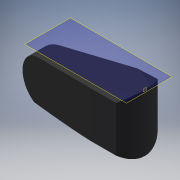
# Autodesk Inventor part: Sample Euph
Saved by Autodesk Inventor 2018 (Build 220112000, 112)
## iProperties
Created: 2018-02-07
Part Number: Sample Euph
Material: Generic
Document SubType Name: Modeling
Designer: owner
Density: 1 g/cm^3
Appearance: Default
Author: owner
Autodesk Inventor part; units mm, degrees
ref_plane "YZ Plane" through (0, 0, 0) normal (1, 0, 0) x (0, 1, 0)
ref_plane "XZ Plane" through (0, 0, 0) normal (0, 1, 0) x (-1, 0, 0)
ref_plane "XY Plane" through (0, 0, 0) normal (0, 0, 1) x (1, 0, 0)
sketch "Sketch1" plane through (0, 0, 0) normal (0, 0, 1) x (1, 0, 0)
  line L0 (171.45, 0) -> (908.05, 0)
  line L1 (0, 0) -> (908.05, 0) construction
  line L2 (908.05, 0) -> (908.05, 457.2)
  arc A0 (145.6057, 340.9409) -> (171.45, 0) centre (171.45, 171.45) ccw
  line L3 (908.05, 457.2) -> (145.6057, 340.9409)
  dimension "d0" = 908.05
  dimension "d2" = 457.2
  dimension "d6" = 342.9
  constraints: 8 end point, 2 horizontal, 2 point on circle, 1 centre point, 1 perpendicular, 1 point on line, 1 tangent
  measures "d0" distance of L1.start L0.end
  measures "d2" distance of L0.end L2.end
  measures "d6" diameter of A0
extrude "Extrusion1" add sketch "Sketch1" against normal blind 330.2
ref_plane "Work Plane1" through (171.45, 473.075, 0) normal (0, -1, 0) x (1, 0, 0)
sketch "Sketch2" plane through (171.45, 473.075, 0) normal (0, -1, 0) x (1, 0, 0)
  line L0 (-171.45, -101.6) -> (466.725, 0)
  line L1 (-171.45, 0) -> (0, 0) projected
  line L2 (-171.45, -101.6) -> (-222.6023, -185.7168)
  line L3 (-222.6023, -185.7168) -> (-171.45, -228.6)
  line L4 (-171.45, -330.2) -> (0, -330.2) projected
  line L5 (-171.45, -330.2) -> (-272.7707, -143.6584)
  line L6 (-272.7707, -143.6584) -> (-171.45, 0)
  line L7 (736.6, 0) -> (736.6, -330.2) projected
  arc A0 (673.1, -330.2) -> (673.1, 0) centre (490.22, -165.1) ccw
  line L8 (-171.45, -228.6) -> (673.1, -330.2)
  line L9 (0, -330.2) -> (732.1184, -387.4806)
  line L10 (732.1184, -387.4806) -> (736.6, -330.2)
  line L11 (0, 0) -> (704.85, 102.8193)
  line L12 (704.85, 102.8193) -> (736.6, 0)
  line L13 (466.725, 0) -> (673.1, 0)
  point P0 (-25.8443, 0)
  point P1 (-25.8443, -330.2)
  constraints: 22 end point, 2 point on circle, 1 centre point, 1 perpendicular, 1 point on line
extrude "Extrusion2" cut sketch "Sketch2" along normal blind 498.475
ref_plane "Work Plane2" through (908.05, 457.2, -165.1) normal (1, 0, 0) x (0, 1, 0)
sketch "Sketch3" plane through (908.05, 457.2, -165.1) normal (1, 0, 0) x (0, 1, 0)
  arc A0 (-403.7389, 165.1) -> (-403.7389, -165.1) centre (-175.5365, 0) ccw
  line L0 (-403.7389, 165.1) -> (-403.7389, -165.1) construction
  line L1 (-403.7389, 165.1) -> (-73.5389, 165.1) construction
  arc A1 (-41.1511, -165.1) -> (-41.1511, 165.1) centre (-351.7698, 0) ccw
  line L2 (-41.1511, 165.1) -> (-41.1511, -165.1) construction
  line L3 (-41.1511, 165.1) -> (289.0489, 165.1) construction
  line L4 (32.9195, -42.2794) -> (0, -311.8659)
  line L5 (0, -311.8659) -> (-365.75, -351.4919)
  line L6 (-365.75, -351.4919) -> (-502.0441, -177.0726)
  line L7 (-502.0441, -177.0726) -> (-491.3232, 238.9194)
  line L8 (-491.3232, 238.9194) -> (-238.6389, 274.5039)
  line L9 (-238.6389, 274.5039) -> (32.9195, 238.9194)
  line L10 (32.9195, 238.9194) -> (32.9195, -42.2794)
  line L11 (-41.1511, 165.1) -> (-403.7389, 165.1)
  line L12 (-41.1511, 165.1) -> (-457.2, 165.1) projected
  line L13 (-403.7389, -165.1) -> (-41.1511, -165.1)
  line L14 (-9.6826, -165.1) -> (-457.2, -165.1) projected
  dimension "d16" = 90
  dimension "d17" = 90
  constraints: 26 end point, 4 point on circle, 2 centre point, 2 collinear, 2 horizontal, 2 perpendicular, 1 vertical
  measures "d16" angle of L0 L1
  measures "d17" angle of L2 L3
extrude "Extrusion3" cut sketch "Sketch3" against normal blind 1038.225
body "Solid1"
